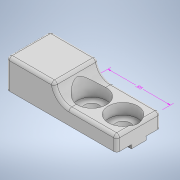
# Autodesk Inventor part: Mount Female V3
Saved by Autodesk Inventor 2020 (Build 240168000, 168)
## iProperties
Created: 2020-01-27
Part Number: Mount Female V3
Material: Generic
Document SubType Name: Modeling
Designer: maple
Density: 1 g/cm^3
Appearance: Default
Author: maple
Autodesk Inventor part; units mm, degrees
ref_plane "YZ Plane" through (0, 0, 0) normal (1, 0, 0) x (0, 1, 0)
ref_plane "XZ Plane" through (0, 0, 0) normal (0, 1, 0) x (-1, 0, 0)
ref_plane "XY Plane" through (0, 0, 0) normal (0, 0, 1) x (1, 0, 0)
sketch "Sketch1" plane through (0, 0, 0) normal (0, 1, 0) x (-1, 0, 0)
  line L0 (0, 0) -> (-38.1, 0)
  line L1 (-38.1, 0) -> (-38.1, -15.24)
  line L2 (-38.1, -15.24) -> (0, -15.24)
  line L3 (0, -15.24) -> (0, 0)
  dimension "d0" = 38.1
  dimension "d1" = 15.24
  constraints: 8 end point, 2 parallel, 1 horizontal, 1 perpendicular
  measures "d0" distance of L2.end L1.end
  measures "d1" distance of L1.end L0.end
extrude "Extrusion1" add sketch "Sketch1" along normal blind 5.08
sketch "Sketch2" plane through (0, 5.08, 0) normal (0, 1, 0) x (1, 0, 0)
  line L0 (0, 0) -> (16.51, 0)
  line L1 (16.51, 0) -> (16.51, 15.24)
  line L2 (16.51, 15.24) -> (0, 15.24)
  line L3 (0, 15.24) -> (0, 0)
  dimension "d4" = 16.51
  dimension "d5" = 15.24
  constraints: 8 end point, 2 parallel, 1 horizontal, 1 perpendicular
  measures "d4" distance of L2.end L1.end
  measures "d5" distance of L1.end L0.end
extrude "Extrusion2" add sketch "Sketch2" along normal blind 5.08
sketch "Sketch3" plane through (0, 0, -15.24) normal (-1, 0, 0) x (0, 0, 1)
  line L0 (0, 10.16) -> (15.24, 10.16) projected
  line L1 (7.62, 10.16) -> (7.62, 8.89)
  line L2 (7.62, 8.89) -> (2.54, 8.89)
  line L3 (2.54, 8.89) -> (2.54, 3.81)
  line L4 (2.54, 3.81) -> (12.7, 3.81)
  line L5 (12.7, 3.81) -> (12.7, 8.89)
  line L6 (12.7, 8.89) -> (7.62, 8.89)
  point P0 (15.24, 0)
  dimension "d8" = 1.27
  dimension "d9" = 5.08
  dimension "d10" = 5.08
  dimension "d11" = 10.16
  dimension "d12" = 90
  dimension "d13" = 5.08
  constraints: 12 end point, 2 perpendicular, 1 horizontal, 1 midpoint, 1 point on line, 1 vertical
  measures "d8" distance of L1.start L1.end
  measures "d9" distance of L1.end L2.end
  measures "d10" distance of L2.end L3.end
  measures "d11" distance of L3.end L4.end
  measures "d12" angle of L4 L3
  measures "d13" distance of L4.end L5.end
extrude "Extrusion3" cut sketch "Sketch3" against normal blind 15.24
sketch "Sketch4" plane through (0, 5.08, 0) normal (0, 1, 0) x (1, 0, 0)
  line L0 (38.1, 0) -> (38.1, 15.24) projected
  line L1 (38.1, 7.62) -> (32.7025, 7.62)
  line L2 (32.7025, 7.62) -> (27.305, 7.62)
  line L3 (27.305, 7.62) -> (21.8948, 7.62)
  point P0 (0, 0)
  dimension "d19" = 5.3975
  dimension "d20" = 5.3975
  dimension "d21" = 180
  dimension "d22" = 5.4102
  dimension "d23" = 180
  constraints: 6 end point, 2 collinear, 1 horizontal, 1 midpoint
  measures "d19" distance of L1.start L1.end
  measures "d20" distance of L1.end L2.end
  measures "d21" angle of L2 L1
  measures "d22" distance of L2.end L3.end
  measures "d23" angle of L3 L2
sketch "Sketch5" plane through (0, 0, 0) normal (0, -1, 0) x (1, 0, 0)
  line L0 (0, -15.24) -> (0, 0) projected
  line L1 (0, -7.62) -> (0, -10.16)
  line L2 (0, -10.16) -> (0, -5.08)
  line L3 (0, -5.08) -> (38.1, -5.08)
  line L4 (38.1, -5.08) -> (38.1, -10.16)
  line L5 (38.1, -10.16) -> (0, -10.16)
  line L6 (0, -10.16) -> (0, -5.08)
  dimension "d31" = 2.54
  dimension "d32" = 5.08
  dimension "d33" = 38.1
  dimension "d34" = 5.08
  constraints: 12 end point, 2 parallel, 2 point on line, 1 horizontal, 1 midpoint, 1 perpendicular
  measures "d31" distance of L1.start L1.end
  measures "d32" distance of L1.end L2.end
  measures "d33" distance of L4.end L5.end
  measures "d34" distance of L3.end L4.end
extrude "Extrusion4" add sketch "Sketch5" along normal blind 1.27
hole "Hole2" at (32.7025, 5.08, -7.62) at (21.8948, 5.08, -7.62) direction (0, -1, 0) diameter 5.08 end through all counterbore diameter 10.16 counterbore depth 3.81
fillet "Fillet1" radius 5.08 1 edges at (16.51, 5.08, -7.62)
fillet "Fillet2" radius 1.016 13 edges at (8.255, 10.16, 0) (8.255, 10.16, -15.24) (0, 5.08, -15.24) (0, 10.16, -7.62) (0, 5.08, 0) (16.51, 10.16, -7.62) (17.9979, 6.5679, 0) (29.845, 5.08, 0) (17.9979, 6.5679, -15.24) (29.845, 5.08, -15.24) (38.1, 5.08, -7.62) (38.1, 2.54, 0) (38.1, 2.54, -15.24)
fillet "Fillet3" radius 0.508 4 edges at (0, 3.81, -7.62) (0, 6.35, -2.54) (0, 6.35, -12.7) (0, 8.89, -7.62)
body "Solid1"
